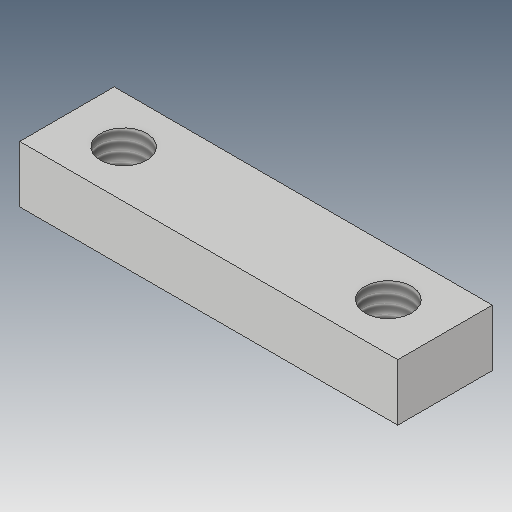
# Autodesk Inventor part: Key1
Saved by Autodesk Inventor 2019.4 (Build 234330000, 330)
## iProperties
Created: 2019-06-16
Part Number: Key1
Material: Generic
Document SubType Name: Modeling
Designer: AzLIer
Density: 1 g/cm^3
Appearance: Default
Mass: 0.271506 g
Surface Area: 3.77355 cm^2
Volume: 0.271506 cm^3
Author: AzLIer
Autodesk Inventor part; units mm, degrees
ref_plane "YZ Plane" through (0, 0, 0) normal (1, 0, 0) x (0, 1, 0)
ref_plane "XZ Plane" through (0, 0, 0) normal (0, 1, 0) x (-1, 0, 0)
ref_plane "XY Plane" through (0, 0, 0) normal (0, 0, 1) x (1, 0, 0)
sketch "スケッチ1" plane through (0, 0, 0) normal (0, 0, 1) x (1, 0, 0)
  line L0 (-10, 1.5) -> (10, 1.5)
  line L1 (10, 1.5) -> (10, -1.5)
  line L2 (10, -1.5) -> (-10, -1.5)
  line L3 (-10, -1.5) -> (-10, 1.5)
  line L4 (-10, 1.5) -> (10, -1.5) construction
  line L5 (10, 1.5) -> (-10, -1.5) construction
  point P0 (0, 0)
  dimension "d0" = 20
  dimension "d1" = 3
  constraints: 12 end point, 2 midpoint, 2 parallel, 1 horizontal, 1 perpendicular
  measures "d0" distance of L1.end L2.end
  measures "d1" distance of L0.end L1.end
extrude "押し出し1" add sketch "スケッチ1" along normal blind 5
sketch "スケッチ2" plane through (-10, 1.5, 0) normal (0, 1, 0) x (1, 0, 0)
  line L0 (0, 0) -> (20, 0) projected
  line L1 (0, 0) -> (0, -5) projected
  line L2 (20, -5) -> (0, -5) projected
  line L3 (20, 0) -> (20, -5) projected
  line L4 (17, -2.5) -> (3, -2.5)
  line L5 (0, 0) -> (0, -5) projected
  point P0 (10, 0)
  point P1 (10, -5)
  point P2 (10, -2.5)
  point P3 (0, -2.5)
  dimension "d4" = 14
  constraints: 3 midpoint, 2 end point, 1 horizontal, 1 horizontal alignment, 1 vertical alignment
  measures "d4" distance of L4.start L4.end
hole "穴1" at (-7, 1.5, 2.5) at (7, 1.5, 2.5) direction (0, -1, 0) diameter 2.459 depth 8.8 tip angle 118 thread size "M3x0.5" class "6H" standard "ISO Metric profile"
